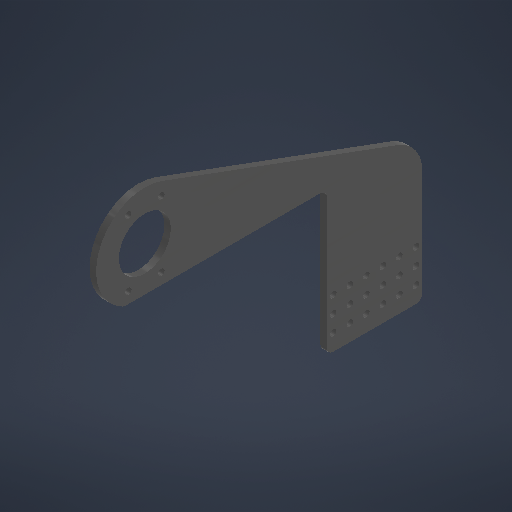
# Autodesk Inventor part: CHAPA FIXAÇÃO DIREITA 2
Saved by Autodesk Inventor 2026 (Build 300175000, 175)
## iProperties
Created: 2026-06-17
Part Number: CHAPA FIXAÇÃO DIREITA 2
Material: Genérico
Document SubType Name: Modeling
Designer: DELL
Density: 1 g/cm^3
Appearance: Cinza escuro
Author: DELL
Autodesk Inventor part; units mm, degrees
ref_plane "YZ Plane" through (0, 0, 0) normal (1, 0, 0) x (0, 1, 0)
ref_plane "XZ Plane" through (0, 0, 0) normal (0, 1, 0) x (-1, 0, 0)
ref_plane "XY Plane" through (0, 0, 0) normal (0, 0, 1) x (1, 0, 0)
sketch "Esboço1" plane through (0, 0, 0) normal (1, 0, 0) x (0, 1, 0)
  line L0 (0, 0) -> (50.8, 0)
  line L1 (50.8, 0) -> (50.8, -86.2)
  line L2 (50.8, -86.2) -> (0, -86.2)
  line L3 (0, -86.2) -> (0, 0)
  dimension "d0" = 50.8
  dimension "d1" = 86.2
  constraints: 8 end point, 2 parallel, 1 horizontal, 1 perpendicular
  measures "d0" distance of L1.end L2.end
  measures "d1" distance of L0.end L1.end
extrude "Extrusão1" add sketch "Esboço1" along normal blind 5
sketch "Esboço2" plane through (5, 0, 0) normal (1, 0, 0) x (0, 0, -1)
  circle A0 centre (5, 12.7) radius 2.5
  circle A1 centre (5, 25.4) radius 2.5
  circle A2 centre (5, 38.1) radius 2.5
  line L0 (0, 50.8) -> (0, 0) projected
  line L1 (86.2, 50.8) -> (0, 50.8) projected
  line L2 (0, 0) -> (86.2, 0) projected
  dimension "d4" = 5
  dimension "d5" = 5
  dimension "d6" = 5
  dimension "d7" = 5
  dimension "d8" = 5
  dimension "d9" = 5
  dimension "d10" = 12.7
  dimension "d11" = 12.7
  dimension "d12" = 12.7
  constraints: 3 centre point
  measures "d4" diameter of A0
  measures "d5" diameter of A1
  measures "d6" diameter of A2
  measures "d7" distance from line of L0 A0.centre
  measures "d8" distance from line of L0 A1.centre
  measures "d9" distance from line of L0 A2.centre
  measures "d10" distance from line of L1 A2.centre
  measures "d11" distance of A2.centre A1.centre
  measures "d12" distance of A1.centre A0.centre
extrude "Extrusão2" cut sketch "Esboço2" against normal blind 6
pattern_linear "Padrão retangular1" count 7 spacing 12.7 along (0, 0, -1) of "Extrusão2"
sketch "Esboço3" plane through (0, 0, 0) normal (-1, 0, 0) x (0, 0, 1)
  line L0 (0, 50.8) -> (0, 0) projected
  line L1 (0, 0) -> (-86.2, 0) projected
  line L2 (0, 50.8) -> (-50.8, 50.8)
  line L3 (-50.8, 50.8) -> (-50.8, 0)
  line L4 (-50.8, 0) -> (0, 0)
  line L5 (0, 0) -> (0, 50.8)
  circle A0 centre (-55.8, 25.4) radius 2.5 projected
  dimension "d19" = 5
  constraints: 8 end point, 2 parallel, 1 horizontal, 1 perpendicular, 1 point on line
  measures "d19" distance from line of A0.centre L3
extrude "Extrusão3" cut sketch "Esboço3" against normal blind 10 contours L0 L1 L3 L2
sketch "Esboço4" plane through (5, 0, 0) normal (1, 0, 0) x (0, 0, -1)
  line L0 (86.2, 0) -> (86.2, 50.8) projected
  line L1 (86.2, 50.8) -> (124.3, 50.8)
  line L2 (124.3, 50.8) -> (124.3, 0)
  line L3 (124.3, 0) -> (86.2, 0)
  line L4 (86.2, 0) -> (86.2, 50.8)
  circle A0 centre (93.9, 25.4) radius 2.5 projected
  circle A1 centre (93.9, 38.1) radius 2.5 projected
  circle A2 centre (106.6, 38.1) radius 2.5 projected
  circle A3 centre (119.3, 38.1) radius 2.5 projected
  circle A4 centre (119.3, 25.4) radius 2.5 projected
  circle A5 centre (106.6, 25.4) radius 2.5 projected
  circle A6 centre (93.9, 12.7) radius 2.5 projected
  circle A7 centre (106.6, 12.7) radius 2.5 projected
  circle A8 centre (119.3, 12.7) radius 2.5 projected
  point P0 (0, 0)
  dimension "d22" = 5
  dimension "d23" = 50.8
  constraints: 8 end point, 2 parallel, 1 horizontal, 1 perpendicular
  measures "d22" distance from line of L2 A4.centre
  measures "d23" distance of L1.end L2.end
extrude "Extrusão4" add sketch "Esboço4" against normal blind 5
sketch "Esboço7" plane through (5, 0, 0) normal (1, 0, 0) x (0, 0, -1)
  line L0 (124.3, 50.8) -> (50.8, 50.8) projected
  line L1 (124.3, 50.8) -> (124.3, 85.9607)
  circle A0 centre (95.7, 85.9607) radius 11.25 projected
  circle A1 centre (-89.125, 144.496) radius 17.5 projected
  circle A2 centre (95.7, 111.3607) radius 2.0193 projected
  circle A3 centre (77.7395, 103.9212) radius 2.0193 projected
  circle A4 centre (95.7, 60.5607) radius 2.0193 projected
  circle A5 centre (113.6605, 68.0002) radius 2.0193 projected
  circle A6 centre (-101.825, 169.896) radius 2.5 projected
  circle A7 centre (-76.425, 169.896) radius 2.5 projected
  circle A8 centre (-76.425, 119.096) radius 2.5 projected
  circle A9 centre (-101.825, 119.096) radius 2.5 projected
  arc A10 (-76.1735, 179.6885) -> (-105.0332, 110.5375) centre (-89.125, 144.496) ccw
  arc A11 (124.3, 85.9607) -> (105.5776, 112.8008) centre (95.7, 85.9607) ccw
  line L2 (50.8, 0) -> (50.8, 50.8) projected
  line L3 (50.8, 50.8) -> (50.8, 110.5375)
  line L4 (50.8, 110.5375) -> (-105.0332, 110.5375)
  line L5 (54.784, 109.5375) -> (24.05, 109.5375) projected
  line L6 (-76.1735, 179.6885) -> (105.5776, 112.8008)
  circle A12 centre (-89.125, 144.496) radius 20
  circle A13 centre (95.7, 85.9607) radius 14.25
  point P0 (0, 0)
  dimension "d36" = 75
  dimension "d37" = 1
  dimension "d38" = 40
  dimension "d39" = 28.5
  constraints: 8 end point, 4 centre point, 4 coincident, 4 point on circle, 3 tangent, 2 vertical, 1 perpendicular
  measures "d36" diameter of A10
  measures "d37" distance between parallel lines of L5 L4
  measures "d38" diameter of A12
  measures "d39" diameter of A13
extrude "Extrusão6" add sketch "Esboço7" against normal blind 5 contours L0 L3 L4 A10 L6 A11 L1
fillet "Arredondamento1" radius 5 4 edges at (2.5, 110.5375, -50.8) (2.5, 110.5375, 105.0332) (2.5, 0, -50.8) (2.5, 0, -124.3)
sketch "Esboço8" plane through (0, 0, 0) normal (-1, 0, 0) x (0, 0, 1)
  circle A0 centre (-95.7, 85.9607) radius 14.25 projected
  circle A1 centre (-113.6605, 68.0002) radius 2.0193 projected
  circle A2 centre (-95.7, 60.5607) radius 2.0193 projected
  circle A3 centre (-95.7, 111.3607) radius 2.0193 projected
  circle A4 centre (-77.7395, 103.9212) radius 2.0193 projected
  point P0 (0, 0)
extrude "Extrusão7" add sketch "Esboço8" against normal blind 5
equation "\"d8\" = d7"
equation "\"d9\" = d8"
equation "\"d11\" = d10"
equation "\"d12\" = d11"
